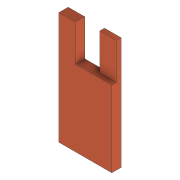
# Autodesk Inventor part: Thermistor
Saved by Autodesk Inventor 2021 (Build 250183000, 183)
## iProperties
Created: 2025-07-03
Part Number: Thermistor
Material: Generic
Document SubType Name: Modeling
Designer: Owner
Density: 1 g/cm^3
Appearance: Default
Author: Owner
Autodesk Inventor part; units mm, degrees
ref_plane "YZ Plane" through (0, 0, 0) normal (1, 0, 0) x (0, 1, 0)
ref_plane "XZ Plane" through (0, 0, 0) normal (0, 1, 0) x (-1, 0, 0)
ref_plane "XY Plane" through (0, 0, 0) normal (0, 0, 1) x (1, 0, 0)
sketch "Sketch1" plane through (0, 0, 0) normal (0, 0, 1) x (1, 0, 0)
  line L0 (-4, 8.5) -> (4, 8.5)
  line L1 (4, 8.5) -> (4, -8.5)
  line L2 (4, -8.5) -> (-4, -8.5)
  line L3 (-4, -8.5) -> (-4, 8.5)
  line L4 (-4, 8.5) -> (4, -8.5) construction
  line L5 (4, 8.5) -> (-4, -8.5) construction
  point P0 (0, 0)
  dimension "d0" = 8
  dimension "d1" = 17
  constraints: 12 end point, 2 midpoint, 2 parallel, 1 horizontal, 1 perpendicular
  measures "d0" distance of L1.end L2.end
  measures "d1" distance of L0.end L1.end
extrude "Extrusion1" add sketch "Sketch1" along normal blind 1.4
sketch "Sketch2" plane through (0, 0, 1.4) normal (0, 0, 1) x (1, 0, 0)
  line L0 (4, 8.5) -> (-4, 8.5) projected
  line L1 (-1.5, 8.5) -> (1.5, 8.5)
  line L2 (1.5, 8.5) -> (1.5, 3)
  line L3 (1.5, 3) -> (-1.5, 3)
  line L4 (-1.5, 3) -> (-1.5, 8.5)
  line L5 (4, -8.5) -> (4, 8.5) projected
  point P0 (0, 0)
  point P1 (1.5, 8.5)
  dimension "d4" = 3
  dimension "d5" = 5.5
  dimension "d6" = 2.5
  constraints: 8 end point, 2 parallel, 1 horizontal, 1 perpendicular, 1 point on line
  measures "d4" distance of L2.end L3.end
  measures "d5" distance of L1.end L2.end
  measures "d6" distance between parallel lines of L5 L2
extrude "Extrusion2" cut sketch "Sketch2" against normal blind 1.4
sketch "Sketch3" plane through (0, 0, 1.4) normal (0, 0, 1) x (1, 0, 0)
  line L0 (4, 8.5) -> (1.5, 8.5) projected
  line L1 (4, -8.5) -> (4, 8.5) projected
  line L2 (1.5, 8.5) -> (4, 8.5)
  line L3 (4, 8.5) -> (4, 3)
  line L4 (4, 3) -> (1.5, 3)
  line L5 (1.5, 3) -> (1.5, 8.5)
  point P0 (0, 0)
  dimension "d9" = 5.5
  constraints: 8 end point, 2 parallel, 1 horizontal, 1 perpendicular, 1 point on line
  measures "d9" distance of L2.end L3.end
extrude "Extrusion3" cut sketch "Sketch3" against normal blind 0.7
body "Solid1"
